Autodesk Fusion 360 part; units mm, degrees
(part 7 of 7)
equation "case_h = 60.0000000 mm" comment "Front height"
equation "case_d = 34.0000000 mm" comment "Rear wiring margin included"
equation "wall = 2.4000000 mm" comment "Structural shell wall"
equation "front_lip = 1.6000000 mm" comment "Front optical lip"
equation "front_depth = 9.5000000 mm" comment "Main front/rear seam"
equation "acrylic_t = 3.1750000 mm" comment "Nominal Amazon 1/8 inch; measure actual sheet"
equation "panel_w = 104.0000000 mm" comment "Shared optical outline"
equation "panel_h = 38.0000000 mm" comment "Shared optical outline"
equation "air_gap = 0.5000000 mm" comment "Rear engraving to white letter tips"
equation "backing_base = 1.6000000 mm" comment "Black printed base"
equation "letter_relief = 0.4000000 mm" comment "White letters above black base"
equation "tray_t = 1.6000000 mm" comment "Optical retainer thickness"
equation "fit = 0.2500000 mm" comment "Nominal mating clearance per side"
equation "m3_hole = 3.6 mm" comment "M3 clearance"
equation "nut_af = 6 mm" comment "Ordinary M3 nut trap"
equation "head_d = 6.8 mm" comment "M3 socket-head counterbore"
equation "head_depth = 3.2000000 mm" comment "Front bearing plane"
equation "led_w = 8.0000000 mm" comment "Separated LED module"
equation "led_h = 8.0000000 mm" comment "Separated LED module"
equation "led_t = 2.0000000 mm" comment "LED module thickness"
equation "led_optical_offset = 1.0000000 mm" comment "Unmeasured emitter center from module front"
equation "text_h = 18.0000000 mm" comment "Reference text height"
equation "switch_w = 8.6000000 mm" comment "DPDT case"
equation "switch_h = 3.1000000 mm" comment "DPDT case depth"
equation "switch_t = 2.7000000 mm" comment "DPDT case front-to-actuator axis"
equation "switch_throw = 2.58 mm" comment "Confirmed: full slot 4 mm minus actuator width 1.42 mm"
equation "actuator_w = 1.4200000 mm" comment "Updated reported actuator width"
equation "actuator_d = 1.42 mm" comment "Confirmed actuator thickness"
equation "actuator_h = 1.8300000 mm" comment "Updated reported actuator height"
equation "reset_y = 54.7000000 mm" comment "Provisional XIAO reset center"
equation "reset_depth = 14.5500000 mm" comment "Provisional XIAO reset center"
equation "reset_tip_x = 113.7000000 mm" comment "Contact tip; 0.2 mm free play to reference button"
equation "reset_stroke = 0.5000000 mm" comment "0.2 free play + 0.3 actuation allowance"
equation "spdt_body_length = 10.5000000 mm" comment "Amazon Tnuocke SS12F15-G5 dimension drawing"
equation "spdt_body_depth = 5.7000000 mm" comment "Listing drawing; axis normal to sign face"
equation "spdt_body_height = 5.5000000 mm" comment "Drawing: flange face to terminal base"
equation "spdt_flange_length = 19.5000000 mm" comment "Drawing; no mounting-hole assumption"
equation "spdt_knob_height = 5.0000000 mm" comment "Drawing"
equation "spdt_knob_envelope = 3.2000000 mm" comment "Conservative square envelope; drawing side dimension 2.9 mm"
equation "spdt_travel = 3.0000000 mm" comment "Nominal family travel, unmeasured; aperture allows 4.7 mm total"
equation "spdt_fit_clearance = 0.3000000 mm" comment "Per side in X and Y; front keeper clearance 0.35 mm"
named bodies: "Front bezel envelope", "Front compression seat", "Front compression seat (1)", "Front compression seat (2)", "Front compression seat (3)", "LED floor", "LED lateral guide", "LED lateral guide (1)", "LED floor (1)", "LED lateral guide (2)", "LED lateral guide (3)", "LED floor (2)", "LED lateral guide (4)", "LED lateral guide (5)", "LED floor (3)", "LED lateral guide (6)", "LED lateral guide (7)", "Shared left datum", "Shared left datum (1)", "Shared lower datum", "Shared lower datum (1)", "Right compliant pad wall", "Right compliant pad wall (1)", "Upper compliant pad wall", "Upper compliant pad wall (1)", "Side tongue root", "Side tongue root (1)", "Side locating tongue", "Side locating tongue (1)", "Upper tongue root", "Upper locating tongue", "Optical clamp boss", "Optical clamp boss (1)", "Clear acrylic sheet", "Black substrate", "Raised letter 0", "Raised letter 2", "Raised letter 3", "Raised letter 5", "Raised letter 6", "Hidden acrylic spacing pad", "Hidden acrylic spacing pad (1)", "Hidden acrylic spacing pad (2)", "Hidden acrylic spacing pad (3)", "Hidden acrylic spacing pad (4)", "Hidden acrylic spacing pad (5)", "Hidden acrylic spacing pad (6)", "Hidden acrylic spacing pad (7)", "Hidden acrylic spacing pad (8)", "Hidden acrylic spacing pad (9)", "Hidden acrylic spacing pad (10)", "Hidden acrylic spacing pad (11)", "Perimeter retainer", "Optical screw ear", "Optical screw ear (1)", "LED pad connection", "LED pad connection (1)", "LED hold-down pad", "LED hold-down pad (1)", "LED pad connection (2)", "LED pad connection (3)", "LED hold-down pad (2)", "LED hold-down pad (3)", "Laminate front spacer", "Laminate rear shim", "Rear housing envelope", "Closure boss", "Battery fence", "Battery fence (1)", "Battery fence (2)", "Battery fence (3)", "Battery bed", "Raised strap lug", "Raised strap lug (1)", "Charger PCB seat", "Charger PCB seat (1)", "Charger PCB seat (2)", "Charger PCB seat (3)", "Charger side fence", "Charger side fence (1)", "Charger insertion stop", "Charger extraction stop", "Charger extraction stop (1)", "XIAO inner spine", "XIAO rear outer cheek", "XIAO rear depth stop", "XIAO lower axial stop", "XIAO upper axial stop", "DPDT rear seat", "DPDT side cheek", "DPDT side cheek (1)", "DPDT axial stop", "DPDT axial stop (1)", "DPDT axial stop (2)", "DPDT axial stop (3)", "Yoke mounting boss", "Reset guide collar", "Reset collar underside gusset", "Reset stop root", "Reset stop root gusset", "Reset inward stop", "Common yoke rail", "Charger yoke arm", "Charger yoke arm (1)", "Charger keeper foot", "Charger keeper foot (1)", "Charger keeper foot (2)", "Charger keeper foot (3)", "Switch yoke arm", "Switch yoke arm (1)", "Switch retaining foot", "Switch retaining foot (1)", "XIAO yoke rail", "Reset stop arm", "Reset stop post", "Reset stop 45 degree brace", "XIAO restraint root", "XIAO front outer restraint", "XIAO restraint root (1)", "XIAO front outer restraint (1)", "Yoke screw pad", "Yoke screw pad (1)", "Reset exterior stem", "Reset captive flange", "Reset contact tip", "Actuator cup blank", "Inner captive flange", "Slider guide neck", "Exterior finger grip", "Battery pouch", "Charger PCB", "Charger USB envelope", "Charger IC envelope", "XIAO PCB", "XIAO USB envelope", "XIAO component envelope", "XIAO reset target", "DPDT body", "DPDT actuator", "DPDT terminal", "DPDT terminal (1)", "DPDT terminal (2)", "DPDT terminal (3)", "DPDT terminal (4)", "DPDT terminal (5)", "LED module", "LED module (1)", "LED module (2)", "LED module (3)", "Closure screw head", "Closure screw shaft", "Closure screw head (1)", "Closure screw shaft (1)", "Closure screw head (2)", "Closure screw shaft (2)", "Closure screw head (3)", "Closure screw shaft (3)", "Optical screw head", "Optical screw shaft", "Optical screw head (1)", "Optical screw shaft (1)", "Yoke screw head", "Yoke screw shaft", "Yoke screw head (1)", "Yoke screw shaft (1)", "M3 nut", "M3 nut (1)", "M3 nut (2)", "M3 nut (3)", "M3 nut (4)", "M3 nut (5)", "M3 nut (6)", "M3 nut (7)", "Charger port cap arm", "Charger port cap arm (1)", "Charger port roof", "XIAO port cap arm", "XIAO port roof", "Slider cap arm", "Slider cap arm (1)", "Slider guide roof", "Reset cap arm", "Reset guide roof", "Charger broad port cap root", "XIAO broad port cap root", "Slider broad port cap root", "Reset broad cap root", "Battery fence corner union", "Full-width keyed corner", "BOOST insulating landing", "BOOST lateral locating fence", "BOOST lateral locating fence (1)", "SIGNAL insulating landing", "SIGNAL lateral locating fence", "SIGNAL lateral locating fence (1)", "Harness strap anchor", "Harness strap anchor (1)", "SPDT rear seat", "SPDT side locating cheek", "SPDT side locating cheek (1)", "SPDT terminal-side shoulder stop", "SPDT terminal-side shoulder stop (1)", "SPDT flange-side stop tied to top wall", "SPDT keeper arm", "SPDT keeper arm (1)", "SPDT keeper pad with 0.35mm axial allowance", "SPDT keeper pad with 0.35mm axial allowance (1)", "SPDT top-opening roof root", "SPDT removable lever-slot roof", "SPDT main body", "SPDT flange envelope", "SPDT solder terminal envelope", "SPDT solder terminal envelope (1)", "SPDT solder terminal envelope (2)", "SPDT lever", "C1 680uF maximum 8x11.5mm"
